Autodesk Fusion 360 part; units mm, degrees
(part 3 of 6)
  line L1595 (39.37, 227.241805) -> (39.405278, 227.100694)
  line L1596 (29.739167, 285.59125) -> (29.562778, 285.555972)
  line L1597 (39.934444, 235.002917) -> (39.934444, 234.897083)
  line L1598 (22.718889, 226.289305) -> (22.577778, 226.430417)
  line L1599 (35.665833, 227.312361) -> (35.771667, 227.241805)
  line L1600 (24.906111, 285.626528) -> (24.835556, 285.59125)
  line L1601 (21.59, 237.613472) -> (21.942778, 237.119583)
  line L1602 (21.942778, 237.119583) -> (22.366111, 236.660972)
  line L1603 (35.983333, 294.763472) -> (35.983333, 293.705139)
  line L1604 (16.016111, 226.889028) -> (15.910278, 226.85375)
  line L1605 (41.874722, 273.490972) -> (40.781111, 273.490972)
  line L1606 (41.345556, 275.325417) -> (41.874722, 273.490972)
  line L1607 (37.853056, 285.732361) -> (37.888333, 285.661805)
  line L1608 (37.888333, 285.661805) -> (37.923611, 285.59125)
  line L1609 (37.923611, 285.59125) -> (38.064722, 285.555972)
  line L1610 (38.205833, 289.754028) -> (38.241111, 289.71875)
  line L1611 (38.205833, 294.834028) -> (38.1, 294.763472)
  line L1612 (29.245278, 251.442361) -> (29.174722, 251.442361)
  line L1613 (38.981944, 242.975694) -> (39.511111, 242.834583)
  line L1614 (38.629167, 243.116805) -> (38.840833, 243.010972)
  line L1615 (27.340278, 295.186805) -> (27.481389, 295.292639)
  line L1616 (36.83, 227.382917) -> (36.583056, 227.312361)
  line L1617 (36.583056, 227.312361) -> (36.5125, 227.277083)
  line L1618 (27.234444, 253.029861) -> (27.305, 252.88875)
  line L1619 (37.817778, 289.648194) -> (37.817778, 289.542361)
  line L1620 (22.366111, 228.899861) -> (22.613056, 228.75875)
  line L1621 (22.613056, 228.75875) -> (22.895278, 228.688194)
  line L1622 (38.770278, 241.211805) -> (39.123056, 241.14125)
  line L1623 (38.452778, 242.481805) -> (38.311667, 242.446528)
  line L1624 (38.311667, 242.446528) -> (38.241111, 242.340694)
  line L1625 (29.845, 235.567361) -> (29.280556, 235.285139)
  line L1626 (33.090556, 242.375972) -> (32.949444, 243.010972)
  line L1627 (32.949444, 243.010972) -> (32.737778, 243.575417)
  line L1628 (20.919722, 289.612917) -> (20.919722, 289.471805)
  line L1629 (23.8125, 289.542361) -> (23.777222, 289.648194)
  line L1630 (39.264167, 237.01375) -> (39.158333, 237.01375)
  line L1631 (28.469167, 250.313472) -> (28.363333, 250.313472)
  line L1632 (29.845, 285.873472) -> (29.845, 285.802917)
  line L1633 (28.539722, 250.313472) -> (28.469167, 250.313472)
  line L1634 (10.724444, 224.772361) -> (10.830278, 224.63125)
  line L1635 (10.830278, 224.63125) -> (10.900833, 224.595972)
  line L1636 (26.740556, 289.754028) -> (26.811111, 289.789305)
  line L1637 (42.192222, 265.130139) -> (41.980556, 265.27125)
  line L1638 (41.980556, 265.27125) -> (41.768889, 265.341805)
  line L1639 (41.768889, 265.341805) -> (41.521944, 265.377083)
  line L1640 (42.192222, 265.130139) -> (42.368611, 264.918472)
  line L1641 (39.511111, 242.834583) -> (38.981944, 242.975694)
  line L1642 (21.2725, 289.824583) -> (21.096111, 289.789305)
  line L1643 (38.452778, 240.329861) -> (38.276389, 240.365139)
  line L1644 (22.577778, 224.137361) -> (22.577778, 224.349028)
  line L1645 (39.334722, 249.07875) -> (39.264167, 249.07875)
  line L1646 (16.121944, 223.255417) -> (16.086667, 223.220139)
  line L1647 (27.481389, 234.826528) -> (26.846389, 234.79125)
  line L1648 (38.276389, 240.365139) -> (38.205833, 240.435694)
  line L1649 (28.610278, 250.34875) -> (28.539722, 250.313472)
  line L1650 (26.67, 289.648194) -> (26.740556, 289.754028)
  line L1651 (27.305, 291.200417) -> (27.269722, 291.270972)
  line L1652 (33.090556, 239.906528) -> (32.949444, 239.306805)
  line L1653 (28.081111, 234.932361) -> (27.481389, 234.826528)
  line L1654 (21.131389, 285.555972) -> (21.237222, 285.555972)
  line L1655 (20.919722, 289.471805) -> (20.919722, 285.90875)
  line L1656 (29.809722, 285.697083) -> (29.739167, 285.59125)
  line L1657 (9.454444, 227.241805) -> (9.419167, 227.030139)
  line L1658 (15.769167, 226.85375) -> (15.910278, 226.85375)
  line L1659 (15.910278, 226.85375) -> (16.016111, 226.889028)
  line L1660 (23.777222, 289.436528) -> (23.8125, 289.542361)
  line L1661 (38.170556, 240.576805) -> (38.205833, 240.682639)
  line L1662 (39.863889, 242.446528) -> (39.722778, 242.72875)
  line L1663 (40.075556, 228.75875) -> (40.181389, 228.75875)
  line L1664 (40.181389, 228.75875) -> (40.251944, 228.829305)
  line L1665 (33.090556, 239.906528) -> (33.161111, 240.541528)
  line L1666 (33.161111, 240.541528) -> (33.196389, 241.14125)
  line L1667 (20.919722, 285.767639) -> (21.025556, 285.626528)
  line L1668 (21.025556, 285.626528) -> (21.131389, 285.555972)
  line L1669 (38.241111, 240.717917) -> (38.276389, 240.753194)
  line L1670 (38.205833, 240.435694) -> (38.170556, 240.576805)
  line L1671 (28.645556, 250.384028) -> (28.610278, 250.34875)
  line L1672 (30.374167, 235.884861) -> (30.868056, 236.237639)
  line L1673 (30.868056, 236.237639) -> (31.361944, 236.660972)
  line L1674 (28.716111, 235.073472) -> (28.081111, 234.932361)
  line L1675 (28.680833, 250.560417) -> (28.645556, 250.384028)
  line L1676 (39.334722, 290.494861) -> (39.334722, 295.43375)
  line L1677 (33.196389, 241.14125) -> (33.161111, 241.77625)
  line L1678 (33.161111, 241.77625) -> (33.090556, 242.375972)
  line L1679 (38.241111, 289.71875) -> (38.276389, 289.612917)
  line L1680 (12.241389, 227.347639) -> (12.170833, 227.312361)
  line L1681 (12.170833, 227.312361) -> (12.100278, 227.206528)
  line L1682 (12.594167, 227.100694) -> (12.558889, 227.206528)
  line L1683 (12.065, 223.325972) -> (12.065, 223.255417)
  line L1684 (12.065, 226.112917) -> (12.065, 223.431805)
  line L1685 (37.923611, 285.59125) -> (37.888333, 285.661805)
  line L1686 (37.888333, 285.661805) -> (37.853056, 285.732361)
  line L1687 (32.914167, 226.959583) -> (32.984722, 226.889028)
  line L1688 (32.984722, 226.889028) -> (33.196389, 226.85375)
  line L1689 (33.231667, 227.382917) -> (32.984722, 227.312361)
  line L1690 (43.991389, 293.740417) -> (39.334722, 289.08375)
  line L1691 (26.846389, 247.49125) -> (26.246667, 247.455972)
  line L1692 (26.246667, 247.455972) -> (25.611667, 247.385417)
  line L1693 (12.558889, 227.206528) -> (12.523611, 227.312361)
  line L1694 (12.523611, 227.312361) -> (12.453056, 227.347639)
  line L1695 (19.438056, 223.184861) -> (19.508611, 223.220139)
  line L1696 (19.508611, 223.220139) -> (19.579167, 223.325972)
  line L1697 (38.064722, 291.553194) -> (38.170556, 291.553194)
  line L1698 (23.142222, 287.743194) -> (23.1775, 287.778472)
  line L1699 (32.984722, 227.312361) -> (32.914167, 227.277083)
  line L1700 (32.914167, 227.277083) -> (32.878889, 227.241805)
  line L1701 (32.878889, 227.241805) -> (32.843611, 227.135972)
  line L1702 (35.454167, 227.382917) -> (33.231667, 227.382917)
  line L1703 (38.276389, 291.482639) -> (38.346944, 291.376805)
  line L1704 (38.170556, 291.553194) -> (38.276389, 291.482639)
  line L1705 (38.064722, 285.555972) -> (37.923611, 285.59125)
  line L1706 (35.806944, 295.292639) -> (35.630556, 295.292639)
  line L1707 (35.630556, 295.292639) -> (35.489444, 295.186805)
  line L1708 (11.288889, 224.807639) -> (12.065, 226.112917)
  line L1709 (10.971389, 224.595972) -> (11.1125, 224.595972)
  line L1710 (11.1125, 224.595972) -> (11.183056, 224.666528)
  line L1711 (35.771667, 227.100694) -> (35.771667, 227.241805)
  line L1712 (35.771667, 227.241805) -> (35.665833, 227.312361)
  line L1713 (22.895278, 287.707917) -> (23.142222, 287.743194)
  line L1714 (37.853056, 285.732361) -> (37.817778, 285.802917)
  line L1715 (12.100278, 227.206528) -> (11.006667, 225.372083)
  line L1716 (12.347222, 227.382917) -> (12.241389, 227.347639)
  line L1717 (37.817778, 285.802917) -> (37.817778, 285.873472)
  line L1718 (35.665833, 227.312361) -> (35.454167, 227.382917)
  line L1719 (39.0525, 226.85375) -> (39.264167, 226.889028)
  line L1720 (39.264167, 226.889028) -> (39.334722, 226.924305)
  line L1721 (5.856111, 227.17125) -> (5.856111, 227.030139)
  line L1722 (8.396111, 227.382917) -> (6.208889, 227.382917)
  line L1723 (39.334722, 226.924305) -> (39.37, 226.994861)
  line L1724 (39.37, 226.994861) -> (39.405278, 227.100694)
  line L1725 (38.170556, 226.85375) -> (39.0525, 226.85375)
  line L1726 (23.212778, 287.81375) -> (23.248056, 287.954861)
  line L1727 (38.241111, 249.466805) -> (38.346944, 249.431528)
  line L1728 (6.208889, 227.382917) -> (6.0325, 227.347639)
  line L1729 (6.0325, 227.347639) -> (5.891389, 227.277083)
  line L1730 (5.891389, 227.277083) -> (5.856111, 227.17125)
  line L1731 (38.170556, 223.431805) -> (38.170556, 226.85375)
  line L1732 (22.083889, 229.570139) -> (22.154444, 229.217361)
  line L1733 (22.154444, 229.217361) -> (22.366111, 228.899861)
  line L1734 (11.006667, 225.372083) -> (9.913056, 227.17125)
  line L1735 (38.170556, 223.255417) -> (38.170556, 223.36125)
  line L1736 (38.170556, 223.36125) -> (38.170556, 223.431805)
  line L1737 (37.923611, 223.114305) -> (38.064722, 223.149583)
  line L1738 (27.163889, 223.643472) -> (26.740556, 223.749305)
  line L1739 (26.740556, 223.749305) -> (26.387778, 223.99625)
  line L1740 (26.387778, 223.99625) -> (26.211389, 224.31375)
  line L1741 (9.454444, 223.220139) -> (9.489722, 223.184861)
  line L1742 (9.489722, 223.184861) -> (9.525, 223.149583)
  line L1743 (37.182778, 261.14375) -> (37.112222, 261.179028)
  line L1744 (38.1, 252.924028) -> (38.1, 249.749028)
  line L1745 (38.346944, 253.20625) -> (38.276389, 253.20625)
  line L1746 (38.276389, 253.20625) -> (38.205833, 253.170972)
  line L1747 (38.205833, 253.170972) -> (38.135278, 253.100417)
  line L1748 (27.269722, 291.270972) -> (27.269722, 291.376805)
  line L1749 (29.280556, 235.285139) -> (29.845, 235.567361)
  line L1750 (29.845, 235.567361) -> (30.374167, 235.884861)
  line L1751 (36.300833, 261.46125) -> (36.300833, 261.531805)
  line L1752 (36.053889, 261.14375) -> (36.159722, 261.14375)
  line L1753 (36.159722, 261.14375) -> (36.265556, 261.214305)
  line L1754 (22.965833, 223.643472) -> (22.789444, 223.467083)
  line L1755 (22.789444, 223.467083) -> (22.5425, 223.290694)
  line L1756 (22.5425, 223.290694) -> (22.225, 223.184861)
  line L1757 (34.572222, 293.352361) -> (34.748611, 293.705139)
  line L1758 (34.748611, 293.705139) -> (34.783889, 294.057917)
  line L1759 (30.832778, 295.080972) -> (30.868056, 295.186805)
  line L1760 (23.142222, 228.723472) -> (22.895278, 228.688194)
  line L1761 (40.357778, 232.992083) -> (40.3225, 232.956805)
  line L1762 (35.806944, 287.707917) -> (37.817778, 287.707917)
  line L1763 (35.806944, 285.873472) -> (35.806944, 287.707917)
  line L1764 (35.595278, 285.555972) -> (35.665833, 285.555972)
  line L1765 (24.553333, 286.049861) -> (24.482778, 285.90875)
  line L1766 (24.482778, 285.90875) -> (24.482778, 285.802917)
  line L1767 (29.950833, 294.79875) -> (30.091944, 294.834028)
  line L1768 (35.454167, 295.080972) -> (35.454167, 294.939861)
  line L1769 (37.994167, 295.292639) -> (35.806944, 295.292639)
  line L1770 (38.311667, 295.045694) -> (38.311667, 295.11625)
  line L1771 (40.357778, 236.484583) -> (40.357778, 236.414028)
  line L1772 (39.758056, 246.397639) -> (38.770278, 246.397639)
  line L1773 (39.405278, 244.95125) -> (39.087778, 244.915972)
  line L1774 (39.440556, 244.95125) -> (39.405278, 244.95125)
  line L1775 (40.146111, 244.457361) -> (40.005, 244.669028)
  line L1776 (40.005, 244.669028) -> (39.793333, 244.845417)
  line L1777 (24.800278, 289.365972) -> (25.646944, 287.884305)
  line L1778 (24.729722, 289.577639) -> (24.765, 289.471805)
  line L1779 (23.741944, 289.71875) -> (23.671389, 289.789305)
  line L1780 (23.671389, 289.789305) -> (23.459722, 289.824583)
  line L1781 (29.386389, 293.705139) -> (29.245278, 293.705139)
  line L1782 (39.334722, 226.924305) -> (39.264167, 226.889028)
  line L1783 (21.695833, 226.818472) -> (21.448889, 226.712639)
  line L1784 (23.565556, 289.295417) -> (23.706667, 289.330694)
  line L1785 (40.251944, 236.625694) -> (40.3225, 236.555139)
  line L1786 (28.716111, 230.557917) -> (28.716111, 230.452083)
  line L1787 (27.058056, 285.59125) -> (26.916944, 285.767639)
  line L1788 (39.0525, 237.154861) -> (39.087778, 237.084305)
  line L1789 (39.017222, 240.329861) -> (39.017222, 237.33125)
  line L1790 (38.452778, 240.329861) -> (39.017222, 240.329861)
  line L1791 (21.060833, 226.254028) -> (20.849167, 225.830694)
  line L1792 (39.440556, 265.553472) -> (39.475833, 265.412361)
  line L1793 (37.817778, 285.873472) -> (37.817778, 285.802917)
  line L1794 (37.817778, 285.802917) -> (37.853056, 285.732361)
  line L1795 (37.817778, 287.707917) -> (37.817778, 285.873472)
  line L1796 (28.610278, 253.52375) -> (28.645556, 253.488472)
  line L1797 (27.340278, 252.641805) -> (27.305, 252.88875)
  line L1798 (27.305, 252.88875) -> (27.234444, 253.029861)
  line L1799 (27.234444, 253.029861) -> (27.128611, 253.135694)
  line L1800 (27.128611, 253.135694) -> (27.022778, 253.170972)
  line L1801 (27.022778, 253.170972) -> (26.916944, 253.20625)
  line L1802 (26.916944, 253.20625) -> (26.387778, 253.20625)
  line L1803 (26.387778, 253.20625) -> (26.387778, 252.077361)
  line L1804 (26.387778, 252.077361) -> (26.881667, 252.077361)
  line L1805 (26.881667, 252.077361) -> (27.022778, 252.112639)
  line L1806 (27.022778, 252.112639) -> (27.128611, 252.147917)
  line L1807 (27.128611, 252.147917) -> (27.199167, 252.183194)
  line L1808 (27.199167, 252.183194) -> (27.305, 252.359583)
  line L1809 (27.305, 252.359583) -> (27.340278, 252.641805)
  line L1810 (35.454167, 295.080972) -> (35.489444, 295.186805)
  line L1811 (24.518056, 253.488472) -> (24.4475, 253.559028)
  line L1812 (28.469167, 289.824583) -> (30.726944, 289.824583)
  line L1813 (42.368611, 264.918472) -> (42.474444, 264.777361)
  line L1814 (37.958889, 289.789305) -> (37.853056, 289.71875)
  line L1815 (37.853056, 289.71875) -> (37.817778, 289.648194)
  line L1816 (28.821944, 231.61625) -> (28.927778, 231.61625)
  line L1817 (28.927778, 231.61625) -> (28.998333, 231.651528)
  line L1818 (20.672778, 295.821805) -> (25.611667, 295.821805)
  line L1819 (29.562778, 285.555972) -> (29.739167, 285.59125)
  line L1820 (40.287222, 236.237639) -> (40.181389, 236.202361)
  line L1821 (40.3225, 236.555139) -> (40.357778, 236.484583)
  line L1822 (38.770278, 246.397639) -> (39.264167, 248.020417)
  line L1823 (39.722778, 295.821805) -> (39.334722, 295.43375)
  line L1824 (27.516667, 248.232083) -> (26.846389, 248.267361)
  line L1825 (26.846389, 248.267361) -> (26.211389, 248.232083)
  line L1826 (29.598056, 228.864583) -> (29.598056, 228.970417)
  line L1827 (31.397222, 231.651528) -> (31.326667, 231.61625)
  line L1828 (37.288611, 261.14375) -> (37.182778, 261.14375)
  line L1829 (24.412222, 235.285139) -> (25.011944, 235.073472)
  line L1830 (25.011944, 235.073472) -> (25.611667, 234.932361)
  line L1831 (30.938611, 295.257361) -> (30.868056, 295.186805)
  line L1832 (6.385278, 225.26625) -> (7.831667, 225.26625)
  line L1833 (16.086667, 226.994861) -> (16.051389, 226.924305)
  line L1834 (39.6875, 232.427639) -> (39.334722, 232.498194)
  line L1835 (18.979444, 241.14125) -> (19.014722, 240.470972)
  line L1836 (19.014722, 240.470972) -> (19.120556, 239.765417)
  line L1837 (27.128611, 252.147917) -> (27.022778, 252.112639)
  line L1838 (11.535833, 232.992083) -> (11.43, 232.639305)
  line L1839 (36.477222, 227.135972) -> (36.477222, 227.030139)
  line L1840 (22.895278, 288.201805) -> (23.106944, 288.166528)
  line L1841 (23.106944, 288.166528) -> (23.1775, 288.13125)
  line L1842 (23.1775, 288.13125) -> (23.212778, 288.025417)
  line L1843 (38.629167, 245.939028) -> (39.899167, 245.939028)
  line L1844 (38.488056, 245.445139) -> (38.629167, 245.939028)
  line L1845 (38.276389, 245.304028) -> (38.346944, 245.304028)
  line L1846 (38.346944, 245.304028) -> (38.4175, 245.339305)
  line L1847 (37.711944, 223.220139) -> (37.7825, 223.149583)
  line L1848 (37.7825, 223.149583) -> (37.923611, 223.114305)
  line L1849 (37.676667, 223.467083) -> (37.676667, 223.396528)
  line L1850 (26.811111, 289.789305) -> (26.916944, 289.824583)
  line L1851 (38.064722, 223.149583) -> (38.170556, 223.255417)
  line L1852 (37.676667, 223.290694) -> (37.711944, 223.220139)
  line L1853 (42.545, 261.955139) -> (42.439167, 261.637639)
  line L1854 (26.387778, 251.689305) -> (26.634722, 251.689305)
  line L1855 (26.387778, 250.560417) -> (26.387778, 251.689305)
  line L1856 (8.501944, 226.85375) -> (8.396111, 226.85375)
  line L1857 (8.396111, 226.85375) -> (6.385278, 226.85375)
  line L1858 (37.817778, 289.542361) -> (37.817778, 288.166528)
  line L1859 (38.064722, 289.824583) -> (37.958889, 289.789305)
  line L1860 (19.014722, 226.324583) -> (19.05, 226.148194)
  line L1861 (26.3525, 290.283194) -> (26.3525, 295.151528)
  line L1862 (25.999722, 229.675972) -> (25.153056, 229.675972)
  line L1863 (39.334722, 295.821805) -> (39.722778, 295.821805)
  line L1864 (37.359167, 261.14375) -> (37.288611, 261.14375)
  line L1865 (39.475833, 265.412361) -> (39.440556, 265.306528)
  line L1866 (40.040278, 236.167083) -> (38.664444, 236.167083)
  line L1867 (37.500278, 261.284861) -> (37.429722, 261.179028)
  line L1868 (30.374167, 235.884861) -> (29.845, 235.567361)
  line L1869 (20.919722, 285.90875) -> (20.919722, 285.767639)
  line L1870 (40.181389, 240.329861) -> (40.040278, 240.329861)
  line L1871 (38.064722, 291.553194) -> (37.994167, 291.588472)
  line L1872 (38.346944, 291.30625) -> (38.346944, 291.376805)
  line L1873 (38.346944, 291.376805) -> (38.276389, 291.482639)
  line L1874 (23.459722, 290.283194) -> (21.484167, 290.283194)
  line L1875 (11.006667, 232.039583) -> (10.724444, 231.792639)
  line L1876 (10.724444, 231.792639) -> (10.442222, 231.61625)
  line L1877 (27.834167, 223.925694) -> (27.587222, 223.749305)
  line L1878 (27.587222, 223.749305) -> (27.375556, 223.67875)
  line L1879 (27.375556, 223.67875) -> (27.163889, 223.643472)
  line L1880 (6.385278, 226.85375) -> (6.385278, 225.760139)
  line L1881 (6.385278, 225.760139) -> (7.831667, 225.760139)
  line L1882 (31.079722, 230.416805) -> (31.044444, 230.416805)
  line L1883 (27.305, 252.359583) -> (27.199167, 252.183194)
  line L1884 (6.385278, 223.643472) -> (6.385278, 225.26625)
  line L1885 (8.431389, 223.643472) -> (6.385278, 223.643472)
  line L1886 (8.5725, 223.643472) -> (8.501944, 223.643472)
  line L1887 (27.199167, 252.183194) -> (27.128611, 252.147917)
  line L1888 (28.645556, 227.206528) -> (28.610278, 227.312361)
  line L1889 (28.610278, 227.312361) -> (28.539722, 227.347639)
  line L1890 (28.539722, 227.347639) -> (28.398611, 227.382917)
  line L1891 (8.113889, 225.689583) -> (8.043333, 225.724861)
  line L1892 (8.043333, 225.724861) -> (7.831667, 225.760139)
  line L1893 (7.831667, 225.26625) -> (8.078611, 225.301528)
  line L1894 (28.151667, 289.40125) -> (28.222222, 289.330694)
  line L1895 (39.511111, 240.329861) -> (40.040278, 240.329861)
  line L1896 (39.511111, 237.295972) -> (39.511111, 240.329861)
  line L1897 (25.611667, 295.821805) -> (20.073056, 290.283194)
  line L1898 (36.089167, 272.57375) -> (36.124444, 272.503194)
  line L1899 (36.124444, 272.503194) -> (36.089167, 272.397361)
  line L1900 (36.089167, 272.397361) -> (36.053889, 272.326805)
  line L1901 (36.053889, 272.326805) -> (35.948056, 272.25625)
  line L1902 (35.948056, 272.25625) -> (35.842222, 272.25625)
  line L1903 (35.842222, 272.25625) -> (35.771667, 272.25625)
  line L1904 (35.771667, 272.25625) -> (35.701111, 272.291528)
  line L1905 (35.701111, 272.291528) -> (35.630556, 272.362083)
  line L1906 (35.630556, 272.362083) -> (35.595278, 272.432639)
  line L1907 (35.595278, 272.432639) -> (35.418889, 272.961805)
  line L1908 (35.418889, 272.961805) -> (34.007778, 272.961805)
  line L1909 (34.007778, 272.961805) -> (33.831389, 272.397361)
  line L1910 (33.831389, 272.397361) -> (33.796111, 272.326805)
  line L1911 (33.796111, 272.326805) -> (33.760833, 272.291528)
  line L1912 (33.760833, 272.291528) -> (33.690278, 272.25625)
  line L1913 (33.690278, 272.25625) -> (33.584444, 272.25625)
  line L1914 (33.584444, 272.25625) -> (33.408056, 272.291528)
  line L1915 (33.408056, 272.291528) -> (33.3375, 272.362083)
  line L1916 (33.3375, 272.362083) -> (33.302222, 272.467917)
  line L1917 (33.302222, 272.467917) -> (33.3375, 272.57375)
  line L1918 (33.3375, 272.57375) -> (33.372778, 272.679583)
  line L1919 (33.372778, 272.679583) -> (34.466389, 276.313194)
  line L1920 (34.466389, 276.313194) -> (34.466389, 276.38375)
  line L1921 (34.466389, 276.38375) -> (34.536944, 276.454305)
  line L1922 (34.536944, 276.454305) -> (34.6075, 276.489583)
  line L1923 (34.6075, 276.489583) -> (34.713333, 276.489583)
  line L1924 (34.713333, 276.489583) -> (34.783889, 276.489583)
  line L1925 (34.783889, 276.489583) -> (34.889722, 276.454305)
  line L1926 (34.889722, 276.454305) -> (34.925, 276.348472)
  line L1927 (34.925, 276.348472) -> (34.995556, 276.242639)
  line L1928 (34.995556, 276.242639) -> (36.089167, 272.644305)
  line L1929 (36.089167, 272.644305) -> (36.089167, 272.57375)
  line L1930 (21.484167, 290.283194) -> (23.459722, 290.283194)
  line L1931 (23.459722, 290.283194) -> (25.011944, 290.283194)
  line L1932 (25.011944, 285.767639) -> (25.964444, 287.390417)
  line L1933 (24.729722, 285.555972) -> (24.835556, 285.59125)
  line L1934 (26.387778, 252.077361) -> (26.387778, 253.20625)
  line L1935 (36.300833, 261.284861) -> (36.336111, 261.390694)
  line L1936 (39.475833, 265.412361) -> (39.440556, 265.553472)
  line L1937 (16.227778, 291.129861) -> (15.980833, 291.129861)
  line L1938 (30.338889, 253.382639) -> (30.338889, 250.525139)
  line L1939 (18.697222, 227.312361) -> (18.273889, 227.382917)
  line L1940 (18.520833, 224.913472) -> (18.979444, 225.089861)
  line L1941 (18.979444, 225.089861) -> (19.332222, 225.407361)
  line L1942 (38.170556, 240.576805) -> (38.205833, 240.435694)
  line L1943 (38.205833, 240.435694) -> (38.276389, 240.365139)
  line L1944 (34.748611, 291.165139) -> (34.783889, 291.235694)
  line L1945 (34.783889, 291.235694) -> (34.819167, 291.30625)
  line L1946 (35.454167, 291.376805) -> (35.454167, 291.235694)
  line L1947 (35.454167, 291.235694) -> (35.524722, 291.094583)
  line L1948 (35.524722, 291.094583) -> (35.665833, 291.059305)
  line L1949 (24.341667, 252.677083) -> (24.765, 251.265972)
  line L1950 (39.123056, 249.043472) -> (39.0525, 248.972917)
  line L1951 (21.942778, 225.513194) -> (21.872222, 225.477917)
  line L1952 (21.872222, 225.477917) -> (21.801667, 225.407361)
  line L1953 (21.801667, 225.407361) -> (21.766389, 225.26625)
  line L1954 (22.154444, 225.548472) -> (22.013333, 225.548472)
  line L1955 (22.895278, 288.201805) -> (21.448889, 288.201805)
  line L1956 (32.349722, 288.272361) -> (32.596667, 288.695694)
  line L1957 (34.113611, 287.460972) -> (33.655, 287.460972)
  line L1958 (33.655, 287.460972) -> (33.513889, 287.460972)
  line L1959 (40.181389, 230.840139) -> (40.287222, 231.122361)
  line L1960 (40.287222, 231.122361) -> (40.3225, 231.404583)
  line L1961 (25.4, 231.93375) -> (25.364722, 231.863194)
  line L1962 (25.788056, 231.827917) -> (25.752778, 231.898472)
  line L1963 (39.899167, 243.187361) -> (40.110833, 242.975694)
  line L1964 (28.328056, 253.559028) -> (28.292778, 253.488472)
  line L1965 (28.292778, 253.488472) -> (28.2575, 253.347361)
  line L1966 (40.146111, 263.260417) -> (40.181389, 262.801805)
  line L1967 (40.181389, 262.801805) -> (40.287222, 262.378472)
  line L1968 (20.849167, 224.666528) -> (20.778611, 224.94875)
  line L1969 (20.778611, 224.94875) -> (20.743333, 225.26625)
  line L1970 (21.942778, 223.643472) -> (21.695833, 223.67875)
  line L1971 (23.106944, 225.336805) -> (23.001111, 225.477917)
  line L1972 (23.001111, 225.477917) -> (22.895278, 225.548472)
  line L1973 (41.416111, 263.119305) -> (41.521944, 263.04875)
  line L1974 (41.521944, 263.507361) -> (41.451389, 263.472083)
  line L1975 (41.451389, 263.472083) -> (41.416111, 263.401528)
  line L1976 (38.241111, 236.555139) -> (38.205833, 236.449305)
  line L1977 (20.531667, 224.031528) -> (20.390556, 224.349028)
  line L1978 (20.390556, 224.349028) -> (20.249444, 224.807639)
  line L1979 (20.249444, 224.807639) -> (20.214167, 225.230972)
  line L1980 (30.832778, 291.235694) -> (30.832778, 291.341528)
  line L1981 (40.181389, 262.801805) -> (40.146111, 263.260417)
  line L1982 (40.357778, 236.414028) -> (40.357778, 236.484583)
  line L1983 (40.357778, 236.484583) -> (40.3225, 236.555139)
  line L1984 (40.3225, 236.555139) -> (40.251944, 236.625694)
  line L1985 (40.251944, 236.625694) -> (40.075556, 236.660972)
  line L1986 (39.616944, 230.34625) -> (39.934444, 230.522639)
  line L1987 (22.225, 223.184861) -> (21.872222, 223.114305)
  line L1988 (21.872222, 223.114305) -> (21.59, 223.149583)
  line L1989 (21.59, 223.149583) -> (21.307778, 223.255417)
  line L1990 (30.938611, 230.381528) -> (30.868056, 230.381528)
  line L1991 (23.777222, 289.648194) -> (23.8125, 289.542361)
  line L1992 (23.8125, 289.542361) -> (23.777222, 289.436528)
  line L1993 (23.777222, 289.436528) -> (23.741944, 289.365972)
  line L1994 (9.913056, 227.17125) -> (11.006667, 225.372083)
  line L1995 (41.839444, 261.179028) -> (42.086389, 261.320139)
  line L1996 (42.086389, 261.320139) -> (42.262778, 261.46125)
  line L1997 (42.262778, 261.46125) -> (42.439167, 261.637639)
  line L1998 (38.276389, 291.129861) -> (38.311667, 291.165139)
  line L1999 (38.311667, 291.165139) -> (38.346944, 291.30625)
  line L2000 (35.771667, 291.059305) -> (37.958889, 291.059305)
  line L2001 (37.711944, 293.246528) -> (37.747222, 293.317083)
  line L2002 (37.747222, 293.317083) -> (37.747222, 293.422917)
  line L2003 (35.983333, 293.175972) -> (37.394444, 293.175972)
  line L2004 (32.349722, 287.108194) -> (32.279167, 287.390417)
  line L2005 (32.279167, 287.390417) -> (32.243889, 287.707917)
  line L2006 (18.803056, 226.677361) -> (18.944167, 226.500972)
  line L2007 (20.849167, 225.830694) -> (20.778611, 225.548472)
  line L2008 (34.360556, 238.742361) -> (34.536944, 239.412639)
  line L2009 (34.536944, 239.412639) -> (34.678056, 240.118194)
  line L2010 (34.678056, 240.118194) -> (34.713333, 240.788472)
  line L2011 (40.498889, 245.656805) -> (39.511111, 248.867083)
  line L2012 (40.534167, 245.515694) -> (40.498889, 245.58625)
  line L2013 (40.498889, 245.58625) -> (40.498889, 245.656805)
  line L2014 (40.287222, 245.304028) -> (40.393056, 245.304028)
  line L2015 (9.913056, 227.17125) -> (9.807222, 227.312361)
  line L2016 (9.807222, 227.312361) -> (9.736667, 227.347639)
  line L2017 (9.736667, 227.347639) -> (9.666111, 227.347639)
  line L2018 (41.945278, 261.884583) -> (42.015833, 262.131528)
  line L2019 (22.507222, 229.429028) -> (22.577778, 229.252639)
  line L2020 (22.577778, 229.252639) -> (22.718889, 229.146805)
  line L2021 (22.718889, 229.146805) -> (22.789444, 229.111528)
  line L2022 (40.040278, 249.537361) -> (40.005, 249.607917)
  line L2023 (38.770278, 241.77625) -> (38.664444, 241.987917)
  line L2024 (38.664444, 241.987917) -> (38.664444, 242.199583)
  line L2025 (29.315833, 285.838194) -> (29.315833, 285.732361)
  line L2026 (29.315833, 289.295417) -> (29.315833, 285.90875)
  line L2027 (31.4325, 228.75875) -> (31.397222, 228.75875)
  line L2028 (27.128611, 251.724583) -> (27.446111, 251.865694)
  line L2029 (24.553333, 253.417917) -> (24.518056, 253.488472)
  line L2030 (25.4, 250.419305) -> (25.435278, 250.489861)
  line L2031 (39.899167, 245.939028) -> (40.040278, 245.480417)
  line L2032 (20.249444, 224.807639) -> (20.390556, 224.349028)
  line L2033 (20.390556, 224.349028) -> (20.531667, 224.031528)
  line L2034 (33.513889, 294.763472) -> (33.690278, 294.763472)
  line L2035 (13.440833, 227.347639) -> (13.581944, 227.382917)
  line L2036 (12.453056, 223.149583) -> (12.523611, 223.220139)
  line L2037 (38.241111, 285.661805) -> (38.205833, 285.626528)
  line L2038 (12.100278, 227.206528) -> (12.170833, 227.312361)
  line L2039 (37.817778, 289.542361) -> (37.817778, 289.648194)
  line L2040 (31.220833, 229.111528) -> (31.397222, 229.07625)
  line L2041 (39.511111, 237.295972) -> (39.475833, 237.119583)
  line L2042 (39.158333, 250.772083) -> (39.123056, 250.807361)
  line L2043 (9.807222, 223.184861) -> (9.666111, 223.114305)
  line L2044 (11.606389, 233.732917) -> (11.606389, 233.344861)
  line L2045 (41.133889, 265.306528) -> (40.886944, 265.130139)
  line L2046 (38.346944, 281.745972) -> (43.991389, 287.390417)
  line L2047 (42.156944, 264.283472) -> (42.051111, 264.424583)
  line L2048 (21.448889, 288.201805) -> (21.448889, 289.295417)
  line L2049 (23.248056, 287.954861) -> (23.212778, 288.025417)
  line L2050 (6.420556, 295.821805) -> (6.561667, 295.821805)
  line L2051 (39.758056, 246.397639) -> (38.770278, 246.397639)
  line L2052 (23.283333, 231.580972) -> (23.389167, 231.475139)
  line L2053 (23.389167, 231.475139) -> (23.495, 231.228194)
  line L2054 (38.135278, 218.034306) -> (42.650833, 222.549861)
  line L2055 (42.650833, 222.549861) -> (43.991389, 222.549861)
  line L2056 (39.969722, 272.57375) -> (39.934444, 272.467917)
  line L2057 (41.063333, 276.313194) -> (40.005, 272.679583)
  line L2058 (35.842222, 261.249583) -> (35.912778, 261.179028)
  line L2059 (35.912778, 261.179028) -> (35.983333, 261.14375)
  line L2060 (35.983333, 261.14375) -> (36.053889, 261.14375)
  line L2061 (31.291389, 280.581805) -> (30.973889, 280.687639)
  line L2062 (30.973889, 280.687639) -> (30.656389, 280.722917)
  line L2063 (32.243889, 258.497917) -> (32.243889, 279.135417)
  line L2064 (30.656389, 256.910417) -> (30.973889, 256.945694)
  line L2065 (9.736667, 231.404583) -> (10.089444, 231.475139)
  line L2066 (10.089444, 231.475139) -> (10.442222, 231.61625)
  line L2067 (10.442222, 231.61625) -> (10.724444, 231.792639)
  line L2068 (10.724444, 231.792639) -> (11.006667, 232.039583)
  line L2069 (34.043056, 223.396528) -> (34.043056, 223.290694)
  line L2070 (34.043056, 226.85375) -> (34.043056, 223.467083)
  line L2071 (23.036389, 226.747917) -> (23.106944, 226.642083)
  line L2072 (41.557222, 276.348472) -> (41.486667, 276.454305)
  line L2073 (41.486667, 276.454305) -> (41.416111, 276.489583)
  line L2074 (32.0675, 223.643472) -> (31.961667, 223.643472)
  line L2075 (40.287222, 262.378472) -> (40.393056, 262.060972)
  line L2076 (41.275, 261.179028) -> (41.028056, 261.249583)
  line L2077 (35.418889, 226.85375) -> (35.665833, 226.889028)
  line L2078 (35.665833, 226.889028) -> (35.736389, 226.924305)
  line L2079 (35.736389, 226.924305) -> (35.771667, 226.994861)
  line L2080 (24.765, 251.265972) -> (24.341667, 252.677083)
  line L2081 (24.341667, 252.677083) -> (23.918333, 251.265972)
  line L2082 (23.918333, 251.265972) -> (24.765, 251.265972)
  line L2083 (1.446389, 281.745972) -> (1.446389, 222.549861)
  line L2084 (1.446389, 222.549861) -> (3.104444, 222.549861)
  line L2085 (20.990278, 223.467083) -> (21.307778, 223.255417)
  line L2086 (21.307778, 223.255417) -> (21.59, 223.149583)
  line L2087 (21.59, 223.149583) -> (21.872222, 223.114305)
  line L2088 (20.214167, 225.230972) -> (20.249444, 224.807639)
  line L2089 (23.106944, 225.195694) -> (23.106944, 225.336805)
  line L2090 (21.484167, 223.749305) -> (21.695833, 223.67875)
  line L2091 (10.900833, 224.595972) -> (10.971389, 224.595972)
  line L2092 (9.913056, 226.112917) -> (10.724444, 224.772361)
  line L2093 (9.913056, 223.467083) -> (9.913056, 226.112917)
  line L2094 (12.523611, 227.312361) -> (12.558889, 227.206528)
  line L2095 (32.102778, 227.347639) -> (31.891111, 227.382917)
  line L2096 (21.942778, 223.643472) -> (22.225, 223.714028)
  line L2097 (34.713333, 240.788472) -> (34.713333, 241.494028)
  line L2098 (34.713333, 241.494028) -> (34.678056, 242.199583)
  line L2099 (34.678056, 242.199583) -> (34.536944, 242.869861)
  line L2100 (27.199167, 284.885694) -> (22.436667, 284.885694)
  line L2101 (33.725556, 284.885694) -> (28.786667, 284.885694)
  line L2102 (14.322778, 295.821805) -> (12.911667, 295.821805)
  line L2103 (43.991389, 288.836805) -> (43.991389, 293.740417)
  line L2104 (39.698083, 284.522333) -> (43.991389, 288.836805)
  line L2105 (39.511111, 250.913194) -> (39.440556, 250.807361)
  line L2106 (23.565556, 229.640694) -> (23.530278, 229.852361)
  line L2107 (23.530278, 229.852361) -> (23.424444, 230.064028)
  line L2108 (23.424444, 230.064028) -> (23.353889, 230.134583)
  line L2109 (13.581944, 223.114305) -> (13.440833, 223.114305)
  line L2110 (41.874722, 264.671528) -> (41.733611, 264.812639)
  line L2111 (31.361944, 231.969028) -> (31.220833, 232.004305)
  line L2112 (27.446111, 285.732361) -> (27.446111, 285.802917)
  line L2113 (26.916944, 285.767639) -> (27.058056, 285.59125)
  line L2114 (38.452778, 245.374583) -> (38.488056, 245.445139)
  line L2115 (38.029444, 245.515694) -> (38.064722, 245.409861)
  line L2116 (38.064722, 245.409861) -> (38.135278, 245.339305)
  line L2117 (38.135278, 245.339305) -> (38.276389, 245.304028)
  line L2118 (6.173611, 223.114305) -> (8.396111, 223.114305)
  line L2119 (5.856111, 223.467083) -> (5.856111, 223.325972)
  line L2120 (5.856111, 223.325972) -> (5.961944, 223.184861)
  line L2121 (35.665833, 289.789305) -> (35.56, 289.824583)
  line L2122 (29.492222, 251.583472) -> (29.421667, 251.477639)
  line L2123 (25.646944, 232.004305) -> (25.576389, 232.004305)
  line L2124 (26.634722, 229.040972) -> (25.788056, 231.827917)
  line L2125 (39.969722, 272.362083) -> (40.040278, 272.291528)
  line L2126 (40.040278, 272.291528) -> (40.216667, 272.25625)
  line L2127 (40.005, 272.679583) -> (39.969722, 272.57375)
  line L2128 (9.454444, 223.220139) -> (9.419167, 223.467083)
  line L2129 (29.915556, 250.454583) -> (29.915556, 250.560417)
  line L2130 (17.321389, 225.407361) -> (17.321389, 226.85375)
  line L2131 (26.3525, 290.283194) -> (25.011944, 290.283194)
  line L2132 (20.531667, 224.031528) -> (20.743333, 223.749305)
  line L2133 (9.877778, 223.220139) -> (9.807222, 223.184861)
  line L2134 (16.121944, 223.467083) -> (16.157222, 223.396528)
  line L2135 (11.43, 232.639305) -> (11.253611, 232.321805)
  line L2136 (38.558611, 251.93625) -> (38.558611, 249.749028)
  line L2137 (21.307778, 223.255417) -> (20.990278, 223.467083)
  line L2138 (20.990278, 223.467083) -> (20.743333, 223.749305)
  line L2139 (20.743333, 223.749305) -> (20.531667, 224.031528)
  line L2140 (17.321389, 226.85375) -> (18.273889, 226.85375)
  line L2141 (35.348333, 285.732361) -> (35.348333, 285.873472)
  line L2142 (39.123056, 250.807361) -> (39.0525, 250.877917)
  line L2143 (31.538333, 280.440694) -> (31.291389, 280.581805)
  line L2144 (8.113889, 225.689583) -> (8.149167, 225.58375)
  line L2145 (8.149167, 225.58375) -> (8.184444, 225.513194)
  line L2146 (19.755556, 237.789861) -> (20.073056, 237.154861)
  line L2147 (20.073056, 237.154861) -> (20.461111, 236.590417)
  line L2148 (20.461111, 236.590417) -> (20.884444, 236.025972)
  line L2149 (20.884444, 236.025972) -> (21.343056, 235.532083)
  line L2150 (16.157222, 223.396528) -> (16.121944, 223.255417)
  line L2151 (33.443333, 286.085139) -> (33.760833, 286.155694)
  line L2152 (33.760833, 286.155694) -> (33.901944, 286.261528)
  line L2153 (43.285833, 281.745972) -> (38.346944, 281.745972)
  line L2154 (41.416111, 263.401528) -> (41.380833, 263.295694)
  line L2155 (12.523611, 223.220139) -> (12.594167, 223.431805)
  line L2156 (12.065, 223.255417) -> (12.135556, 223.184861)
  line L2157 (7.3025, 233.52125) -> (7.337778, 233.168472)
  line L2158 (7.337778, 233.168472) -> (7.443611, 232.815694)
  line L2159 (7.443611, 232.815694) -> (7.584722, 232.498194)
  line L2160 (7.584722, 232.498194) -> (7.796389, 232.180694)
  line L2161 (38.241111, 242.340694) -> (38.205833, 242.164305)
  line L2162 (38.664444, 242.199583) -> (38.664444, 242.305417)
  line L2163 (23.530278, 231.122361) -> (23.565556, 231.051805)
  line L2164 (23.565556, 231.051805) -> (23.600833, 231.051805)
  line L2165 (42.474444, 263.507361) -> (42.368611, 263.542639)
  line L2166 (42.368611, 263.542639) -> (42.2275, 263.542639)
  line L2167 (42.545, 262.202083) -> (42.545, 263.189861)
  line L2168 (38.276389, 289.507083) -> (38.276389, 289.612917)
  line L2169 (38.276389, 289.612917) -> (38.241111, 289.71875)
  line L2170 (42.545, 263.36625) -> (42.545, 263.189861)
  line L2171 (41.345556, 276.489583) -> (41.239722, 276.489583)
  line L2172 (41.239722, 276.489583) -> (41.133889, 276.454305)
  line L2173 (35.983333, 291.588472) -> (37.994167, 291.588472)
  line L2174 (34.783889, 291.412083) -> (34.819167, 291.30625)
  line L2175 (34.819167, 291.30625) -> (34.783889, 291.235694)
  line L2176 (34.783889, 291.235694) -> (34.748611, 291.165139)
  line L2177 (34.748611, 291.165139) -> (34.642778, 291.094583)
  line L2178 (34.642778, 291.094583) -> (34.536944, 291.059305)
  line L2179 (34.536944, 291.059305) -> (34.395833, 291.094583)
  line L2180 (34.395833, 291.094583) -> (34.29, 291.200417)
  line L2181 (34.29, 291.200417) -> (33.090556, 292.823194)
  line L2182 (33.090556, 292.823194) -> (32.526111, 292.823194)
  line L2183 (32.526111, 292.823194) -> (32.526111, 291.376805)
  line L2184 (32.526111, 291.376805) -> (32.490833, 291.165139)
  line L2185 (32.490833, 291.165139) -> (32.455556, 291.094583)
  line L2186 (32.455556, 291.094583) -> (32.385, 291.059305)
  line L2187 (32.385, 291.059305) -> (32.279167, 291.059305)
  line L2188 (32.279167, 291.059305) -> (32.138056, 291.094583)
  line L2189 (32.138056, 291.094583) -> (32.0675, 291.165139)
  line L2190 (32.0675, 291.165139) -> (32.032222, 291.235694)
  line L2191 (32.032222, 291.235694) -> (31.996944, 291.30625)
  line L2192 (31.996944, 291.30625) -> (31.996944, 291.412083)
  line L2193 (31.996944, 291.412083) -> (31.996944, 294.939861)
  line L2194 (31.996944, 294.939861) -> (32.032222, 295.080972)
  line L2195 (32.032222, 295.080972) -> (32.0675, 295.186805)
  line L2196 (32.0675, 295.186805) -> (32.208611, 295.292639)
  line L2197 (32.208611, 295.292639) -> (32.385, 295.292639)
  line L2198 (32.385, 295.292639) -> (33.478611, 295.292639)
  line L2199 (33.478611, 295.292639) -> (33.901944, 295.222083)
  line L2200 (33.901944, 295.222083) -> (34.325278, 295.045694)
  line L2201 (34.325278, 295.045694) -> (34.572222, 294.763472)
  line L2202 (34.572222, 294.763472) -> (34.748611, 294.445972)
  line L2203 (34.748611, 294.445972) -> (34.783889, 294.057917)
  line L2204 (34.783889, 294.057917) -> (34.748611, 293.705139)
  line L2205 (34.748611, 293.705139) -> (34.572222, 293.352361)
  line L2206 (34.572222, 293.352361) -> (34.219444, 292.999583)
  line L2207 (34.219444, 292.999583) -> (33.760833, 292.823194)
  line L2208 (33.760833, 292.823194) -> (34.713333, 291.517917)
  line L2209 (34.713333, 291.517917) -> (34.748611, 291.482639)
  line L2210 (34.748611, 291.482639) -> (34.783889, 291.412083)
  line L2211 (39.934444, 230.522639) -> (40.181389, 230.840139)
  line L2212 (9.419167, 227.030139) -> (9.454444, 227.241805)
  line L2213 (39.334722, 295.43375) -> (39.334722, 290.494861)
  line L2214 (23.459722, 289.295417) -> (23.565556, 289.295417)
  line L2215 (27.022778, 252.112639) -> (26.881667, 252.077361)
  line L2216 (31.291389, 295.010417) -> (31.291389, 295.11625)
  line L2217 (31.291389, 295.11625) -> (31.220833, 295.222083)
  line L2218 (29.845, 228.723472) -> (29.739167, 228.723472)
  line L2219 (23.918333, 251.265972) -> (24.341667, 252.677083)
  line L2220 (22.225, 223.714028) -> (22.401389, 223.819861)
  line L2221 (20.390556, 226.148194) -> (20.284722, 225.689583)
  line L2222 (20.284722, 225.689583) -> (20.214167, 225.230972)
  line L2223 (21.9075, 227.382917) -> (21.413611, 227.277083)
  line L2224 (21.413611, 227.277083) -> (21.096111, 227.100694)
  line L2225 (24.235833, 281.745972) -> (27.375556, 284.885694)
  line L2226 (16.086667, 284.885694) -> (12.946944, 281.745972)
  line L2227 (14.499167, 256.945694) -> (14.781389, 256.910417)
  line L2228 (28.222222, 289.330694) -> (28.151667, 289.40125)
  line L2229 (26.916944, 253.20625) -> (27.022778, 253.170972)
  line L2230 (9.736667, 227.347639) -> (9.807222, 227.312361)
  line L2231 (33.937222, 241.811528) -> (33.9725, 241.14125)
  line L2232 (33.9725, 241.14125) -> (33.937222, 240.50625)
  line L2233 (33.937222, 240.50625) -> (33.831389, 239.835972)
  line L2234 (33.831389, 239.835972) -> (33.690278, 239.200972)
  line L2235 (33.690278, 239.200972) -> (33.478611, 238.60125)
  line L2236 (33.478611, 238.60125) -> (33.231667, 237.96625)
  line L2237 (33.231667, 237.96625) -> (32.914167, 237.401805)
  line L2238 (32.914167, 237.401805) -> (32.526111, 236.872639)
  line L2239 (32.526111, 236.872639) -> (32.102778, 236.37875)
  line L2240 (32.102778, 236.37875) -> (31.644167, 235.884861)
  line L2241 (31.644167, 235.884861) -> (31.150278, 235.461528)
  line L2242 (31.150278, 235.461528) -> (30.585833, 235.10875)
  line L2243 (30.585833, 235.10875) -> (30.021389, 234.79125)
  line L2244 (30.021389, 234.79125) -> (29.421667, 234.509028)
  line L2245 (29.421667, 234.509028) -> (28.786667, 234.297361)
  line L2246 (28.786667, 234.297361) -> (28.151667, 234.15625)
  line L2247 (28.151667, 234.15625) -> (27.516667, 234.085694)
  line L2248 (27.516667, 234.085694) -> (26.846389, 234.050417)
  line L2249 (26.846389, 234.050417) -> (26.211389, 234.085694)
  line L2250 (26.211389, 234.085694) -> (25.541111, 234.15625)
  line L2251 (25.541111, 234.15625) -> (24.906111, 234.297361)
  line L2252 (24.906111, 234.297361) -> (24.271111, 234.509028)
  line L2253 (24.271111, 234.509028) -> (23.671389, 234.79125)
  line L2254 (23.671389, 234.79125) -> (23.106944, 235.10875)
  line L2255 (23.106944, 235.10875) -> (22.577778, 235.461528)
  line L2256 (22.577778, 235.461528) -> (22.048611, 235.884861)
  line L2257 (22.048611, 235.884861) -> (21.59, 236.37875)
  line L2258 (21.59, 236.37875) -> (21.166667, 236.872639)
  line L2259 (21.166667, 236.872639) -> (20.813889, 237.401805)
  line L2260 (20.813889, 237.401805) -> (20.496389, 237.96625)
  line L2261 (20.496389, 237.96625) -> (20.214167, 238.60125)
  line L2262 (20.214167, 238.60125) -> (20.0025, 239.200972)
  line L2263 (20.0025, 239.200972) -> (19.861389, 239.835972)
  line L2264 (19.861389, 239.835972) -> (19.790833, 240.50625)
  line L2265 (19.790833, 240.50625) -> (19.755556, 241.14125)
  line L2266 (19.755556, 241.14125) -> (19.790833, 241.811528)
  line L2267 (19.790833, 241.811528) -> (19.861389, 242.446528)
  line L2268 (19.861389, 242.446528) -> (20.0025, 243.116805)
  line L2269 (20.0025, 243.116805) -> (20.214167, 243.716528)
  line L2270 (20.214167, 243.716528) -> (20.496389, 244.31625)
  line L2271 (20.496389, 244.31625) -> (20.813889, 244.880694)
  line L2272 (20.813889, 244.880694) -> (21.166667, 245.445139)
  line L2273 (21.166667, 245.445139) -> (21.59, 245.939028)
  line L2274 (21.59, 245.939028) -> (22.048611, 246.397639)
  line L2275 (22.048611, 246.397639) -> (22.577778, 246.820972)
  line L2276 (22.577778, 246.820972) -> (23.106944, 247.209028)
  line L2277 (23.106944, 247.209028) -> (23.671389, 247.526528)
  line L2278 (23.671389, 247.526528) -> (24.271111, 247.773472)
  line L2279 (24.271111, 247.773472) -> (24.906111, 247.985139)
  line L2280 (24.906111, 247.985139) -> (25.541111, 248.161528)
  line L2281 (25.541111, 248.161528) -> (26.211389, 248.232083)
  line L2282 (26.211389, 248.232083) -> (26.846389, 248.267361)
  line L2283 (26.846389, 248.267361) -> (27.516667, 248.232083)
  line L2284 (27.516667, 248.232083) -> (28.151667, 248.161528)
  line L2285 (28.151667, 248.161528) -> (28.786667, 247.985139)
  line L2286 (28.786667, 247.985139) -> (29.421667, 247.773472)
  line L2287 (29.421667, 247.773472) -> (30.021389, 247.526528)
  line L2288 (30.021389, 247.526528) -> (30.585833, 247.209028)
  line L2289 (30.585833, 247.209028) -> (31.150278, 246.820972)
  line L2290 (31.150278, 246.820972) -> (31.644167, 246.397639)
  line L2291 (31.644167, 246.397639) -> (32.102778, 245.939028)
  line L2292 (32.102778, 245.939028) -> (32.526111, 245.445139)
  line L2293 (32.526111, 245.445139) -> (32.914167, 244.880694)
  line L2294 (32.914167, 244.880694) -> (33.231667, 244.31625)
  line L2295 (33.231667, 244.31625) -> (33.478611, 243.716528)
  line L2296 (33.478611, 243.716528) -> (33.690278, 243.116805)
  line L2297 (33.690278, 243.116805) -> (33.831389, 242.446528)
  line L2298 (33.831389, 242.446528) -> (33.937222, 241.811528)
  line L2299 (34.572222, 226.85375) -> (35.418889, 226.85375)
  line L2300 (34.572222, 223.431805) -> (34.572222, 226.85375)
  line L2301 (34.536944, 223.255417) -> (34.572222, 223.36125)
  line L2302 (34.219444, 293.84625) -> (34.113611, 293.634583)
  line L2303 (34.113611, 293.634583) -> (34.007778, 293.52875)
  line L2304 (41.133889, 276.454305) -> (41.098611, 276.38375)
  line L2305 (41.098611, 276.38375) -> (41.063333, 276.313194)
  line L2306 (41.5925, 276.242639) -> (41.557222, 276.348472)
  line L2307 (38.276389, 285.873472) -> (38.241111, 285.661805)
  line L2308 (28.680833, 227.030139) -> (28.680833, 227.135972)
  line L2309 (28.680833, 227.135972) -> (28.645556, 227.206528)
  line L2310 (28.680833, 224.701805) -> (28.680833, 227.030139)
  line L2311 (4.550833, 222.549861) -> (9.454444, 222.549861)
  line L2312 (10.900833, 222.549861) -> (15.804444, 222.549861)
  line L2313 (42.2275, 263.542639) -> (42.368611, 263.542639)
  line L2314 (12.241389, 227.347639) -> (12.347222, 227.382917)
  line L2315 (18.238611, 225.407361) -> (17.321389, 225.407361)
  line L2316 (31.220833, 295.222083) -> (31.150278, 295.292639)
  line L2317 (40.710556, 263.754305) -> (40.675278, 263.260417)
  line L2318 (33.831389, 239.835972) -> (33.937222, 240.50625)
  line L2319 (33.937222, 240.50625) -> (33.9725, 241.14125)
  line L2320 (23.1775, 287.778472) -> (23.142222, 287.743194)
  line L2321 (23.142222, 287.743194) -> (22.895278, 287.707917)
  line L2322 (22.895278, 287.707917) -> (21.448889, 287.707917)
  line L2323 (38.170556, 223.36125) -> (38.170556, 223.255417)
  line L2324 (9.525, 223.149583) -> (9.489722, 223.184861)
  line L2325 (43.991389, 293.740417) -> (39.334722, 289.08375)
  line L2326 (36.935833, 281.745972) -> (39.698083, 284.522333)
  line L2327 (7.831667, 225.760139) -> (8.043333, 225.724861)
  line L2328 (8.043333, 225.724861) -> (8.113889, 225.689583)
  line L2329 (40.569444, 261.743472) -> (40.393056, 262.060972)
  line L2330 (25.752778, 231.898472) -> (25.7175, 231.969028)
  line L2331 (25.7175, 231.969028) -> (25.646944, 232.004305)
  line L2332 (23.495, 231.157639) -> (23.530278, 231.122361)
  line L2333 (23.106944, 231.61625) -> (23.283333, 231.580972)
  line L2334 (32.138056, 244.669028) -> (31.75, 245.198194)
  line L2335 (31.75, 245.198194) -> (31.361944, 245.656805)
  line L2336 (13.335, 223.184861) -> (13.264444, 223.325972)
  line L2337 (40.146111, 249.466805) -> (40.075556, 249.502083)
  line L2338 (25.435278, 250.560417) -> (25.4, 250.630972)
  line L2339 (25.223611, 250.313472) -> (25.294167, 250.313472)
  line L2340 (25.294167, 250.313472) -> (25.364722, 250.34875)
  line L2341 (25.364722, 250.34875) -> (25.4, 250.419305)
  line L2342 (12.135556, 223.184861) -> (12.206111, 223.149583)
  line L2343 (12.206111, 223.149583) -> (12.311944, 223.114305)
  line L2344 (12.065, 223.431805) -> (12.065, 223.325972)
  line L2345 (30.585833, 281.745972) -> (33.725556, 284.885694)
  line L2346 (35.136667, 284.885694) -> (31.996944, 281.745972)
  line L2347 (8.078611, 225.301528) -> (8.113889, 225.336805)
  line L2348 (8.113889, 225.336805) -> (8.149167, 225.372083)
  line L2349 (8.149167, 225.372083) -> (8.184444, 225.513194)
  line L2350 (15.980833, 291.129861) -> (20.672778, 295.821805)
  line L2351 (31.079722, 291.059305) -> (31.185556, 291.094583)
  line L2352 (25.611667, 234.932361) -> (26.246667, 234.826528)
  line L2353 (26.246667, 234.826528) -> (26.846389, 234.79125)
  line L2354 (39.511111, 240.329861) -> (39.511111, 237.295972)
  line L2355 (39.899167, 242.234861) -> (39.828611, 241.917361)
  line L2356 (39.828611, 241.917361) -> (39.6875, 241.705694)
  line L2357 (39.405278, 241.599861) -> (39.123056, 241.599861)
  line L2358 (39.6875, 241.705694) -> (39.546389, 241.635139)
  line L2359 (39.546389, 241.635139) -> (39.405278, 241.599861)
  line L2360 (26.634722, 228.75875) -> (26.67, 228.829305)
  line L2361 (26.67, 228.829305) -> (26.67, 228.899861)
  line L2362 (35.771667, 226.994861) -> (35.771667, 227.030139)
  line L2363 (35.771667, 227.030139) -> (35.771667, 227.100694)
  line L2364 (35.806944, 289.648194) -> (35.736389, 289.754028)
  line L2365 (35.736389, 289.754028) -> (35.665833, 289.789305)
  line L2366 (8.501944, 223.643472) -> (8.431389, 223.643472)
  line L2367 (8.748889, 223.396528) -> (8.748889, 223.467083)
  line L2368 (8.748889, 223.467083) -> (8.713611, 223.537639)
  line L2369 (23.671389, 250.419305) -> (23.777222, 250.842639)
  line L2370 (41.416111, 276.489583) -> (41.345556, 276.489583)
  line L2371 (42.686111, 272.644305) -> (41.5925, 276.242639)
  line L2372 (25.893889, 223.784583) -> (26.176111, 223.467083)
  line L2373 (26.176111, 223.467083) -> (26.634722, 223.220139)
  line L2374 (26.634722, 223.220139) -> (27.163889, 223.114305)
  line L2375 (25.576389, 231.087083) -> (25.999722, 229.675972)
  line L2376 (8.043333, 231.93375) -> (8.325556, 231.686805)
  line L2377 (8.325556, 231.686805) -> (8.643056, 231.545694)
  line L2378 (8.643056, 231.545694) -> (8.995833, 231.439861)
  line L2379 (8.995833, 231.439861) -> (9.383889, 231.369305)
  line L2380 (22.577778, 230.98125) -> (22.5425, 231.157639)
  line L2381 (22.86, 230.699028) -> (22.754167, 230.734305)
  line L2382 (11.253611, 232.321805) -> (11.006667, 232.039583)
  line L2383 (41.204444, 222.549861) -> (36.724167, 218.034306)
  line L2384 (36.724167, 218.034306) -> (31.785278, 218.034306)
  line L2385 (31.785278, 218.034306) -> (36.300833, 222.549861)
  line L2386 (34.043056, 261.284861) -> (34.219444, 261.849305)